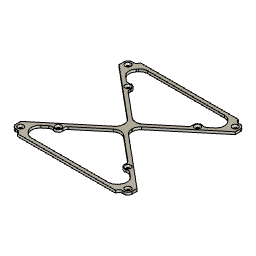
frame-regular (Autodesk Fusion 360 design; units mm, degrees)
Autodesk Fusion 360 part; units mm, degrees
sketch "Sketch1" plane through (0, 0, 0) normal (0, 0, 1) x (1, 0, 0)
  line L0 (0, 0) -> (150, 0)
  line L1 (150, 0) -> (150, 150)
  line L2 (150, 150) -> (0, 150)
  line L3 (0, 150) -> (0, 0)
  dimension "d1" = 150
  dimension "d2" = 150
  constraint horizontal L0
  constraint vertical L1
  constraint horizontal L2
  constraint vertical L3
  constraint coincident L0.start L3.end
  measures "d1" distance of L0.start L0.end
  measures "d2" distance of L0.start L2.end
extrude "Extrude1" add sketch "Sketch1" along normal blind 3
sketch "Sketch2" plane through (0, 0, 3) normal (0, 0, 1) x (-1, 0, 0)
  line L0 (0, -150) -> (0, 0)
  line L1 (0, 0) -> (-150, 0)
  line L2 (-150, 0) -> (-150, -150)
  line L3 (-150, -150) -> (0, -150)
  arc A0 (-4, -9) -> (-9, -4) centre (-9, -9) ccw
  line L4 (0, 0) -> (-15, 0)
  line L5 (-11, -4) -> (-9, -4)
  line L6 (-4, -9) -> (-4, -15)
  line L7 (-4, -15) -> (0, -15)
  line L8 (0, 0) -> (0, -15)
  arc A1 (-15, 0) -> (-11, -4) centre (-11, 0) ccw
  point P0 (-15, 0)
  point P1 (-15, -4)
  point P2 (-9, -4)
  point P3 (-4, -9)
  point P4 (-4, -15)
  point P5 (0, -15)
  dimension "d8" = 15
  dimension "d11" = 5
  dimension "d12" = 4
  dimension "d13" = 4
  dimension "d14" = 15
  dimension "d222" = 4
  constraint coincident L1 P0
  constraint coincident L0 P5
  constraint coincident P2 A0.end
  constraint coincident P3 A0.start
  constraint coincident L0.end L1.start
  constraint coincident P0 L4.end
  constraint tangent A0 L5
  constraint coincident P4 L6.end
  constraint tangent A0 L6
  constraint coincident P5 L7.end
  constraint perpendicular L0 L7
  constraint tangent L5 A1
  measures "d8" distance of L0.end L4.end
  measures "d11" radius of A0
  measures "d12" distance of P0 P1
  measures "d13" distance of P4 P5
  measures "d14" distance of L0.end P5
  measures "d222" radius of A1
sketch "Sketch3" plane through (0, 0, 3) normal (0, 0, 1) x (-1, 0, 0)
  line L0 (-150, -150) -> (0, -150)
  line L1 (0, -150) -> (0, 0)
  line L2 (0, 0) -> (-150, 0)
  line L3 (-150, 0) -> (-150, -150)
  line L4 (0, -75) -> (-70, -75)
  line L5 (-70, -75) -> (-70, -70)
  line L6 (-70, -70) -> (-4, -15)
  line L7 (-4, -15) -> (0, -15)
  line L8 (0, -15) -> (0, -75)
  point P0 (0, -75)
  point P1 (-70, -75)
  point P2 (-70, -70)
  point P3 (0, -15)
  dimension "d25" = 70
  dimension "d27" = 5
  dimension "d50" = 4
  dimension "d51" = 15
  dimension "d52" = 4
  constraint midpoint L1 P0
  constraint coincident P0 L4.start
  constraint coincident P1 L4.end
  constraint perpendicular L1 L4
  constraint coincident P2 L5.end
  constraint perpendicular L4 L5
  constraint coincident L1 P3
  constraint coincident P3 L7.end
  measures "d25" distance of P0 P1
  measures "d27" distance of P1 P2
  measures "d50" horizontal distance of L1.end L6.end
  measures "d51" vertical distance of L1.end L6.end
  measures "d52" distance of L6.end P3
sketch "Sketch4" plane through (0, 0, 3) normal (0, 0, 1) x (-1, 0, 0)
  line L0 (-150, -150) -> (0, -150)
  line L1 (0, 0) -> (-150, 0)
  line L2 (-76.5085, -70) -> (-75, -70)
  line L3 (-75, -70) -> (-75, -4)
  line L4 (-75, -4) -> (-23.4306, -4)
  line L5 (-150, 0) -> (-150, -150)
  line L6 (0, -150) -> (0, 0)
  line L7 (-12.7248, -16.8469) -> (-23.4306, -4)
  line L8 (-12.7248, -16.8469) -> (-76.5085, -70)
  line L9 (-70, -70) -> (-4, -15)
  point P0 (-76.5085, -70)
  point P1 (-75, -70)
  point P2 (-23.4306, -4)
  point P3 (-75, -4)
  point P4 (-12.7248, -16.8469)
  point P5 (-70, -70)
  dimension "d37" = 75
  dimension "d38" = 70
  dimension "d40" = 4
  dimension "d42" = 75
  dimension "d43" = 4
  dimension "d60" = 5
  constraint coincident P0 L2.start
  constraint coincident P1 L2.end
  constraint coincident P3 L3.end
  constraint coincident P2 L4.end
  constraint coincident P4 L7.start
  constraint parallel L8 L9
  constraint perpendicular L7 L8
  constraint perpendicular L2 L3
  measures "d37" horizontal distance of L1.start P1
  measures "d38" vertical distance of L1.start P1
  measures "d40" distance of L1 P2
  measures "d42" horizontal distance of L1.start P3
  measures "d43" distance of L1 P3
ref_plane "WorkPlane2" through (0, 75, 0) normal (0, 1, 0) x (0, 0, 1)
ref_plane "WorkPlane1" through (75, 0, 0) normal (1, 0, 0) x (0, 1, 0)
extrude "Extrude5" cut sketch "Sketch2" sketch "Sketch3" sketch "Sketch4" against normal blind 3 contours L0 L1 A0 L4 L5 L6 L7 L8 A1 of sketch 2 contours L1 L4 L5 L6 L7 L8 of sketch 3 contours L3 L4 L7 L8
sketch "Sketch5" plane through (0, 0, 3) normal (0, 0, 1) x (-1, 0, 0)
  line L0 (0, 0) -> (0, -15)
  point P0 (-9.5, -9.5)
  dimension "d67" = 9.5
  dimension "d68" = 9.5
  measures "d67" vertical distance of P0 L0.start
  measures "d68" distance of P0 L0
hole "Hole1" at (9.5, 9.5, 3) direction (0, 0, -1) diameter 3.2 depth 3 tip angle 180 countersink diameter 7 countersink angle 90
sketch "Sketch15" plane through (0, 0, 3) normal (0, 0, 1) x (-1, 0, 0)
  circle A0 centre (-75, -75) radius 60.1041 construction
  line L0 (-32.5, -32.5) -> (-117.5, -32.5) construction
  line L1 (-117.5, -32.5) -> (-117.5, -117.5) construction
  line L2 (-117.5, -117.5) -> (-32.5, -117.5) construction
  line L3 (-32.5, -117.5) -> (-32.5, -32.5) construction
  circle A1 centre (-32.5, -32.5) radius 4.5
  point P0 (-75, -75)
  point P1 (-32.5, -32.5)
  dimension "d200" = 75
  dimension "d201" = 75
  dimension "d204" = 85
  dimension "d205" = 9
  dimension "d206" = 85
  constraint coincident P0 A0.centre
  constraint horizontal L0
  constraint vertical L1
  constraint horizontal L2
  constraint vertical L3
  constraint coincident A0 L1.end
  constraint coincident A0 P1
  constraint coincident A0 L2.end
  constraint coincident P1 L0.start
  measures "d200" horizontal distance of P0 origin
  measures "d201" vertical distance of P0 origin
  measures "d204" distance of P1 L0.end
  measures "d205" diameter of A1
  measures "d206" distance of L0.end L1.end
extrude "Extrude9" add sketch "Sketch15" against normal blind 3
hole "Hole7" at (32.5, 32.5, 3) direction (0, 0, -1) diameter 3.2 depth 3 tip angle 180 countersink diameter 7 countersink angle 90
fillet "Fillet8" radius 10 2 edges at (12.7248, 16.8469, 1.5) (23.4306, 4, 1.5)
fillet "Fillet8" radius 5 2 edges at (28.6712, 30.1356, 1.5) (35.5161, 35.8396, 1.5)
mirror "Mirror20" about plane through (75, 0, 0) normal (1, 0, 0) of "Extrude5", "Hole1", "Extrude9", "Hole7", "Fillet8"
mirror "Mirror21" about plane through (0, 75, 0) normal (0, 1, 0) of "Extrude5", "Hole1", "Extrude9", "Hole7", "Fillet8", "Mirror20"
fillet "Fillet15" radius 10 6 edges at (75, 68.7429, 1.5) (80, 80, 1.5) (80, 70, 1.5) (75, 81.2571, 1.5) (70, 70, 1.5) (70, 80, 1.5)
equation "d1 = length_cube"
equation "d2 = length_cube"
equation "length_cube = 150 mm"
equation "thickness = 3 mm"
equation "d5 = thickness"
equation "length_cornerstone = 15 mm"
equation "d8 = length_cornerstone"
equation "distance_corner_cornerstone = 4 mm"
equation "fillet_cornerstone = 5 mm"
equation "d11 = fillet_cornerstone"
equation "d12 = distance_corner_cornerstone"
equation "d13 = distance_corner_cornerstone"
equation "d14 = length_cornerstone"
equation "d17 = length_cube / 2"
equation "d20 = length_cube / 2"
equation "height_centerpiece = 10 mm"
equation "width_centerpiece = 10 mm"
equation "d25 = ( length_cube - width_centerpiece ) / 2"
equation "d27 = height_centerpiece / 2"
equation "d37 = length_cube / 2"
equation "d38 = ( length_cube - height_centerpiece ) / 2"
equation "d40 = distance_corner_cornerstone"
equation "d42 = length_cube / 2"
equation "d43 = distance_corner_cornerstone"
equation "d50 = distance_corner_cornerstone"
equation "d51 = length_cornerstone"
equation "d52 = distance_corner_cornerstone"
equation "d53 = -thickness"
equation "d67 = ( length_cornerstone - distance_corner_cornerstone ) / 2 + distance_corner_cornerstone"
equation "d68 = ( length_cornerstone - distance_corner_cornerstone ) / 2 + distance_corner_cornerstone"
equation "radius_inner_wheel = 46 mm"
equation "radius_outer_wheel = 55 mm"
equation "d200 = length_cube / 2"
equation "d201 = length_cube / 2"
equation "d207 = -thickness"
equation "d222 = distance_corner_cornerstone"
